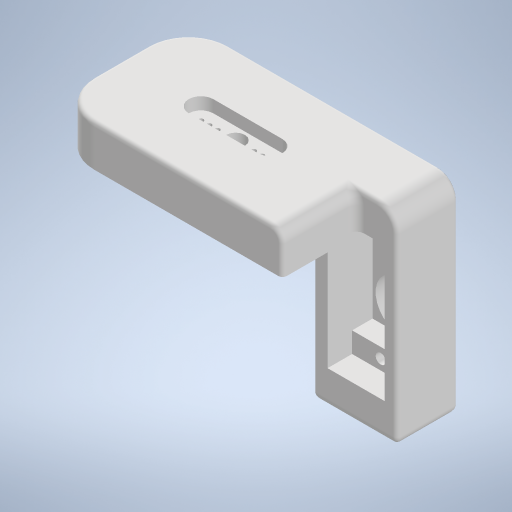
# Autodesk Inventor part: KLESCE
Saved by Autodesk Inventor 2024 (Build 280153000, 153)
## iProperties
Created: 2023-09-14
Part Number: KLESCE
Material: Generic
Document SubType Name: Modeling
Designer: jebes windows
Density: 1 g/cm^3
Appearance: Default
Author: jebes windows
## iProperties of the stored document KLESCE_3DPrint.ipt
Created: 2023-09-14
Part Number: KLESCE_3DPrint
Material: Generic
Document SubType Name: Modeling
Designer: jebes windows
Density: 1 g/cm^3
Appearance: Default
Author: jebes windows
Autodesk Inventor part; units mm, degrees
ref_plane "YZ Plane" through (0, 0, 0) normal (1, 0, 0) x (0, 1, 0)
ref_plane "XZ Plane" through (0, 0, 0) normal (0, 1, 0) x (-1, 0, 0)
ref_plane "XY Plane" through (0, 0, 0) normal (0, 0, 1) x (1, 0, 0)
ref_plane "Work Plane1" through (0, 0, 0) normal (0, 0, 1) x (1, 0, 0)
sketch "Sketch1" plane through (0, 0, 0) normal (0, 0, 1) x (1, 0, 0)
  line L0 (14.1592, 1.9969) -> (2.2091, 2.6499) projected
  arc A0 (2.2091, 2.6499) -> (-2.209, 2.65) centre (0, -0.0001) ccw projected
  line L1 (-2.209, 2.65) -> (-14.1591, 1.997) projected
  arc A1 (-14.1591, 1.997) -> (-14.1591, -1.997) centre (-14.05, 0) ccw projected
  line L2 (-14.1591, -1.997) -> (-2.209, -2.65) projected
  arc A2 (-2.209, -2.65) -> (2.2091, -2.6501) centre (0, -0.0001) ccw projected
  line L3 (2.2091, -2.6501) -> (14.1592, -1.9971) projected
  arc A3 (14.1592, -1.9971) -> (14.1592, 1.9969) centre (14.05, -0.0001) ccw projected
  circle A4 centre (12.45, -0.0001) radius 0.6 projected
  circle A5 centre (14.45, -0.0001) radius 0.6 projected
  circle A6 centre (10.45, -0.0001) radius 0.6 projected
  circle A7 centre (8.45, -0.0001) radius 0.6 projected
  circle A8 centre (6.45, -0.0001) radius 0.6 projected
  circle A9 centre (4.45, -0.0001) radius 0.6 projected
  circle A10 centre (0, -0.0001) radius 2.3 projected
  circle A11 centre (-4.45, 0) radius 0.6 projected
  circle A12 centre (-6.45, 0) radius 0.6 projected
  circle A13 centre (-8.45, 0) radius 0.6 projected
  circle A14 centre (-10.45, 0) radius 0.6 projected
  circle A15 centre (-12.45, 0) radius 0.6 projected
  circle A16 centre (-14.45, 0) radius 0.6 projected
  line L4 (28, -16.5001) -> (-28, -16.5001)
  line L5 (-28, -16.5001) -> (-28, 16.4999)
  line L6 (-28, 16.4999) -> (28, 16.4999)
  line L7 (28, 16.4999) -> (28, -16.5001)
  line L8 (28, -16.5001) -> (-28, 16.4999) construction
  line L9 (-28, -16.5001) -> (28, 16.4999) construction
  line L10 (-15.2779, 6.1803) -> (17.7736, 5.5193)
  point P0 (0, 0)
  dimension "d0" = 56
  dimension "d1" = 33
  constraints: 14 end point, 2 midpoint, 2 parallel, 1 horizontal, 1 perpendicular
  measures "d0" distance of L5.end L6.end
  measures "d1" distance of L4.end L5.end
extrude "Extrusion1" add sketch "Sketch1" along normal blind 10 contours A3 L3 A2 L2 A1 L1 A0 L0 | A4 | A5 | A6 | A14 | A15 | A16 | L4 L5 L6 L7
fillet "Fillet1" radius 10 2 edges at (-28, 16.4999, 5) (-28, -16.5001, 5)
sketch "Sketch5" plane through (28, 16.4999, 10) normal (0, 1, 0) x (1, 0, 0)
  line L0 (0, 0) -> (10, 0)
  line L1 (10, 0) -> (10, 50)
  line L2 (10, 50) -> (-10, 50)
  line L3 (-10, 50) -> (-10, 0)
  line L4 (-46, 0) -> (-46, 10) projected
  line L5 (0, 0) -> (-46, 0) projected
  line L6 (0, 10) -> (0, 0) projected
  line L7 (0, 10) -> (-46, 10) projected
  point P0 (-28, 10)
  point P1 (-10, 0)
  point P2 (-10, 10)
  point P3 (0, 0)
  dimension "d9" = 10
  dimension "d10" = 50
  dimension "d11" = 20
  dimension "d12" = 18
  dimension "d13" = 40
  constraints: 8 end point, 3 perpendicular, 1 horizontal, 1 point on line
  measures "d9" distance of L0.start L0.end
  measures "d10" distance of L0.end L1.end
  measures "d11" distance of L1.end L2.end
  measures "d12" distance from line of point (-28, 10) L3
  measures "d13" distance from line of point (-28, 10) L2
extrude "Extrusion2" add sketch "Sketch5" against normal blind 15 contours L6 L7 L3 L2 L1 L0
sketch "Sketch7" plane through (28, 1.4999, 10) normal (0, -1, 0) x (1, 0, 0)
  line L0 (-7, -36.5) -> (7, -36.5)
  line L1 (7, -36.5) -> (7, -13.5)
  line L2 (7, -13.5) -> (-7, -13.5)
  line L3 (-7, -13.5) -> (-7, -36.5)
  line L4 (-7, -36.5) -> (7, -13.5) construction
  line L5 (7, -36.5) -> (-7, -13.5) construction
  line L6 (-10, -50) -> (10, -50) projected
  line L7 (10, -50) -> (10, 0) projected
  point P0 (-28, -10)
  point P1 (0, -25)
  dimension "d16" = 14
  dimension "d17" = 23
  dimension "d18" = 25
  dimension "d19" = 10
  constraints: 12 end point, 2 midpoint, 2 parallel, 1 horizontal, 1 perpendicular
  measures "d16" distance of L2.end L1.end
  measures "d17" distance of L1.end L0.end
  measures "d18" distance from line of L6 point (0, -25)
  measures "d19" distance from line of L7 point (0, -25)
extrude "Extrusion3" cut sketch "Sketch7" against normal blind 11
sketch "Sketch8" plane through (28, 12.4999, 10) normal (0, -1, 0) x (1, 0, 0)
  line L0 (7, -13.5) -> (7, -36.5) projected
  line L1 (-7, -13.5) -> (7, -13.5) projected
  line L2 (-7, -36.5) -> (-7, -13.5) projected
  line L3 (7, -36.5) -> (-7, -36.5) projected
  circle A0 centre (0, -30.5) radius 6.25
  circle A1 centre (0, -24.25) radius 3.25
  line L4 (7, -36.5) -> (-7, -36.5) projected
  point P0 (-28, -10)
  point P1 (0, -36.5)
  point P2 (0, -36.5)
  point P3 (0, -36.5)
  point P4 (-3.1383, -25.095)
  point P5 (-1.75, -36.5)
  point P6 (1.75, -36.5)
  point P7 (3.1382, -25.095)
  dimension "d22" = 12.5
  dimension "d23" = 6.5
  dimension "d24" = 6
  constraints: 3 midpoint, 2 vertical alignment, 1 centre point, 3 other
  measures "d23" diameter of A1
  measures "d24" distance of point (0, -36.5) point (0, -30.5)
extrude "Extrusion4" cut sketch "Sketch8" against normal blind 11 contours L3 A0 A1 | A1 A0 | A0 A1
sketch "Sketch9" plane through (28, 1.4999, 10) normal (0, -1, 0) x (1, 0, 0)
  arc A0 (-3.1383, -25.095) -> (-1.75, -36.5) centre (0, -30.5) ccw projected
  arc A1 (3.1382, -25.095) -> (-3.1383, -25.095) centre (0, -24.25) ccw projected
  arc A2 (1.75, -36.5) -> (3.1382, -25.095) centre (0, -30.5) ccw projected
  line L0 (7, -36.5) -> (1.75, -36.5) projected
  line L1 (7, -13.5) -> (7, -36.5) projected
  line L2 (-7, -13.5) -> (7, -13.5) projected
  line L3 (-7, -36.5) -> (-7, -13.5) projected
  line L4 (-1.75, -36.5) -> (-7, -36.5) projected
  line L5 (-7, -13.5) -> (7, -13.5) projected
  line L6 (7, -13.5) -> (7, -36.5) projected
  line L7 (7, -36.5) -> (-7, -36.5) projected
  line L8 (-7, -36.5) -> (-7, -13.5) projected
  line L9 (0, -10) -> (0, 0) projected
  line L10 (-10, -10) -> (0, -10) projected
  line L11 (-10, -10) -> (-10, -50) projected
  line L12 (-10, -50) -> (10, -50) projected
  line L13 (10, -50) -> (10, 0) projected
  line L14 (10, 0) -> (0, 0) projected
  line L15 (-7, -36.5) -> (-7, -41.5)
  line L16 (-7, -41.5) -> (7, -41.5)
  line L17 (7, -41.5) -> (7, -36.5)
  line L18 (7, -13.5) -> (7, -8.5)
  line L19 (7, -8.5) -> (-7, -8.5)
  line L20 (-7, -8.5) -> (-7, -13.5)
  circle A3 centre (0, -39) radius 1.25
  circle A4 centre (0, -11) radius 1.25
  point P0 (-28, -10)
  point P1 (7, -39)
  dimension "d27" = 5
  dimension "d28" = 5
  dimension "d29" = 2.5
  dimension "d30" = 2.5
  dimension "d31" = 28
  dimension "d32" = 7
  dimension "d33" = 7
  dimension "d34" = 19.5
  constraints: 12 end point, 3 perpendicular, 2 centre point, 2 vertical, 1 horizontal, 1 midpoint
  measures "d27" distance of L7.end L15.end
  measures "d28" distance of L5.end L18.end
  measures "d29" diameter of A3
  measures "d30" diameter of A4
  measures "d31" distance of A3.centre A4.centre
  measures "d32" distance of point (7, -39) A3.centre
  measures "d33" distance from line of L18 A4.centre
  measures "d34" distance of A0.centre A4.centre
extrude "Extrusion5" cut sketch "Sketch9" against normal blind 6 contours L7 L0 L17 L16 L15 L4 | L20 L10 A4 L9 L19 L18 L2 | L20 L19 L9 A4 L10 | A4 L9 L10 | L10 L9 A4 | A3
sketch "Sketch10" plane through (28, 7.4999, 10) normal (0, -1, 0) x (1, 0, 0)
  line L0 (7, -41.5) -> (-7, -41.5) projected
  line L1 (7, -36.5) -> (7, -41.5) projected
  line L2 (-7, -36.5) -> (7, -36.5) projected
  line L3 (-7, -41.5) -> (-7, -36.5) projected
  line L4 (-7, -8.5) -> (7, -8.5) projected
  line L5 (-7, -13.5) -> (-7, -8.5) projected
  line L6 (7, -13.5) -> (-7, -13.5) projected
  line L7 (7, -8.5) -> (7, -13.5) projected
  circle A0 centre (0, -39) radius 1.25
  circle A1 centre (0, -11) radius 1.25
  point P0 (-28, -10)
  point P1 (7, -39)
  dimension "d37" = 2.5
  dimension "d38" = 2.5
  dimension "d39" = 28
  dimension "d40" = 7
  dimension "d41" = 25.5
  dimension "d42" = 25.5
  constraints: 2 centre point, 1 midpoint
  measures "d37" diameter of A0
  measures "d38" diameter of A1
  measures "d39" distance of A0.centre A1.centre
  measures "d40" distance of point (7, -39) A0.centre
  measures "d41" distance from line of L6 A0.centre
  measures "d42" distance from line of L2 A1.centre
extrude "Extrusion6" cut sketch "Sketch10" against normal blind 5 contours A0 | A1
fillet "Fillet2" radius 5 1 edges at (38, 8.9999, 10)
fillet "Fillet3" radius 3 1 edges at (28, -7.5001, 10)
fillet "Fillet4" radius 1 9 edges at (36.5355, 16.4999, 8.5355) (7.5, 16.4999, 10) (-25.071, 13.571, 10) (-28, -0.0001, 10) (-25.071, -13.5711, 10) (3.5, -16.5001, 10) (27.1214, -16.5001, 9.1213) (28, -16.5001, 3.5) (38, 16.4999, -17.5)
fillet "Fillet5" radius 1 4 edges at (36.5355, 1.4999, 8.5355) (26.5, 1.4999, 10) (30.5, 1.4999, 10) (38, 1.4999, -17.5)
fillet "Fillet6" radius 2 6 edges at (37.7071, 1.7928, -40) (27.5, 1.4999, -40) (37.7071, 16.2071, -40) (27.5, 16.4999, -40) (38, 8.9999, -40) (18, 8.9999, -40)
sketch "Sketch12" plane through (0, 0, 10) normal (0, 0, 1) x (1, 0, 0)
  circle A0 centre (-8.45, 0) radius 0.6 projected
  circle A1 centre (-8.45, 0) radius 3
  circle A2 centre (8.45, -0.0001) radius 0.6 projected
  circle A3 centre (8.45, -0.0001) radius 3
  line L0 (-8.4663, 2.9999) -> (8.45, 2.9999)
  line L1 (-8.45, -3) -> (8.45, -3.0001)
  point P0 (0, 0)
  dimension "d58" = 6
  dimension "d59" = 6
  constraints: 4 end point, 4 point on circle, 3 tangent, 2 centre point, 2 coincident, 1 horizontal
  measures "d58" diameter of A1
  measures "d59" diameter of A3
extrude "Extrusion8" cut sketch "Sketch12" against normal blind 3
fillet "Fillet7" radius 5 1 edges at (18, 8.9999, 0)
fillet "Fillet8" radius 2 2 edges at (15.5, 1.4999, 0) (19.5, 1.4999, 0)
fillet "Fillet9" radius 2 3 edges at (27.8026, 1.4999, 8.0705) (26.1588, 1.8585, 9.7672) (28, 1.4999, 4.25)
body "Solid1"
